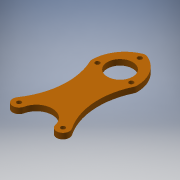
# Autodesk Inventor part: Part69
Saved by Autodesk Inventor 2017 SP1 (Build 210196100, 196)
## iProperties
Created: 2018-01-30
Part Number: Part69
Material: Aluminum 6061
Document SubType Name: Modeling
Designer: Ben
Density: 2.7 g/cm^3
Appearance: Orange
Mass: 68.2139 g
Surface Area: 113.002 cm^2
Volume: 25.2644 cm^3
Author: Ben
Autodesk Inventor part; units mm, degrees
ref_plane "YZ Plane" through (0, 0, 0) normal (1, 0, 0) x (0, 1, 0)
ref_plane "XZ Plane" through (0, 0, 0) normal (0, 1, 0) x (-1, 0, 0)
ref_plane "XY Plane" through (0, 0, 0) normal (0, 0, 1) x (1, 0, 0)
sketch "Sketch1" plane through (0, 0, 0) normal (0, 1, 0) x (-1, 0, 0)
  circle A0 centre (0, 0) radius 14.2875
  line L0 (143.7805, 15.875) -> (-143.7805, 15.875) construction
  line L1 (0, 0) -> (0, 15.875) construction
  line L2 (0, 15.875) -> (0, 88.9254) construction
  line L3 (24.6957, 88.9254) -> (-24.6957, 88.9254) construction
  line L4 (0, 113.6211) -> (0, 64.2297) construction
  circle A1 centre (24.6957, 88.9254) radius 2.4892
  circle A2 centre (-24.6957, 88.9254) radius 2.4892
  circle A3 centre (0, 64.2297) radius 2.4892 construction
  circle A4 centre (0, 113.6211) radius 2.4892 construction
  circle A5 centre (0, 0) radius 50.8 construction
  line L5 (143.7805, -34.925) -> (-143.7805, -34.925) construction
  line L6 (0, 0) -> (0, -34.925) construction
  circle A6 centre (19.05, 6.35) radius 2.54
  circle A7 centre (-19.05, 6.35) radius 2.54
  circle A8 centre (0, -22.225) radius 2.54
  line L7 (19.05, 6.35) -> (-19.05, 6.35) construction
  arc A9 (-2.4454, -28.0852) -> (2.4454, -28.0852) centre (0, -22.225) ccw
  arc A10 (-24.7931, 9.059) -> (-25.4, 6.3466) centre (-19.05, 6.35) ccw
  arc A11 (25.4, 6.3466) -> (24.7931, 9.059) centre (19.05, 6.35) ccw
  arc A12 (30.6963, 84.8535) -> (24.7931, 9.059) centre (94.1678, 41.783) ccw
  arc A13 (-24.7931, 9.059) -> (-30.6963, 84.8535) centre (-94.1678, 41.783) ccw
  arc A14 (2.4454, -28.0852) -> (25.4, 6.3466) centre (-11.9308, 6.3664) ccw
  arc A15 (-25.4, 6.3466) -> (-2.4454, -28.0852) centre (11.9308, 6.3664) ccw
  line L8 (12.3733, -7.1438) -> (20.6222, -11.9063) construction
  arc A16 (-17.6059, 90.4493) -> (-30.6963, 84.8535) centre (-24.6957, 88.9254) ccw
  arc A17 (30.6963, 84.8535) -> (17.6059, 90.4493) centre (24.6957, 88.9254) ccw
  arc A18 (-17.6059, 90.4493) -> (17.6059, 90.4493) centre (0, 94.2334) ccw
  line L9 (-17.4625, 41.783) -> (17.4625, 41.783) construction
  circle A19 centre (0, 88.9254) radius 12.7 construction
  point P0 (0, 6.35)
  dimension "d0" = 28.575
  dimension "d1" = 15.875
  dimension "d3" = 4.9784
  dimension "d4" = 88.9254
  dimension "d5" = 101.6
  dimension "d7" = 50.8
  dimension "d8" = 5.08
  dimension "d9" = 9.525
  dimension "d10" = 38.1
  dimension "d12" = 6.35
  dimension "d18" = 28.575
  dimension "d19" = 9.525
  dimension "d20" = 60
  dimension "d23" = 34.925
  dimension "d25" = 4.7625
  dimension "d26" = 34.925
  dimension "d27" = 25.4
  constraints: 23 point on circle, 20 end point, 19 centre point, 12 coincident, 10 equal radius, 10 tangent, 5 midpoint, 5 point on line, 4 horizontal, 2 equal length, 2 perpendicular, 2 vertical, 1 line through centre, 3 other
  measures "d1" distance of L1.start L1.end
  measures "d3" diameter of A1
  measures "d4" distance of L2.end point (0, 0)
  measures "d5" diameter of A5
  measures "d7" distance between parallel lines of L0 L5
  measures "d8" diameter of A6
  measures "d9" distance between parallel lines of L0 L7
  measures "d10" distance of L7.start L7.end
  measures "d12" radius of A9
  measures "d18" distance from line of L7 A8.centre
  measures "d19" distance of L8.start L8.end
  measures "d20" angle of L6 L8
  measures "d23" distance of L4.end L3.start
  measures "d25" radial gap between concentric circles of A1 A17
  measures "d26" distance of L9.start L9.end
  measures "d27" diameter of A19
extrude "Extrusion1" add sketch "Sketch1" along normal blind 6.35
body "Solid1"
